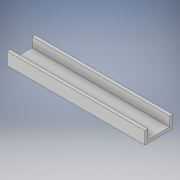
# Autodesk Inventor part: ArmProto1.2
Saved by Autodesk Inventor 2017 (Build 210142000, 142)
## iProperties
Created: 2017-09-30
Part Number: ArmProto1.2
Material: Generic
Document SubType Name: Modeling
Designer: User
Density: 1 g/cm^3
Appearance: Default
Author: User
Autodesk Inventor part; units mm, degrees
ref_plane "YZ Plane" through (0, 0, 0) normal (1, 0, 0) x (0, 1, 0)
ref_plane "XZ Plane" through (0, 0, 0) normal (0, 1, 0) x (-1, 0, 0)
ref_plane "XY Plane" through (0, 0, 0) normal (0, 0, 1) x (1, 0, 0)
sketch "Sketch1" plane through (0, 0, 0) normal (1, 0, 0) x (0, 1, 0)
  line L0 (0, 0) -> (25.4, 0)
  line L1 (25.4, 0) -> (25.4, -57.15)
  line L2 (25.4, -57.15) -> (0, -57.15)
  line L3 (0, -57.15) -> (0, 0)
  line L4 (25.4, -6.35) -> (6.35, -6.35)
  line L5 (6.35, -6.35) -> (6.35, -50.8)
  line L6 (6.35, -50.8) -> (25.4, -50.8)
  line L7 (25.4, -50.8) -> (25.4, -6.35)
  dimension "d0" = 25.4
  dimension "d1" = 57.15
  dimension "d2" = 19.05
  dimension "d3" = 44.45
  dimension "d4" = 6.35
  constraints: 16 end point, 4 parallel, 2 horizontal, 2 perpendicular, 1 point on line
  measures "d0" distance of L1.end L2.end
  measures "d1" distance of L0.end L1.end
  measures "d2" distance of L5.end L6.end
  measures "d3" distance of L4.end L5.end
  measures "d4" distance between parallel lines of L0 L4
extrude "Extrusion1" add sketch "Sketch1" along normal blind 279.4 contours L0 L1 L4 L5 L6 L2 L3
body "Solid1"
